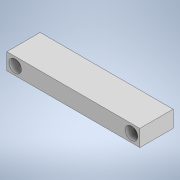
# Autodesk Inventor part: 3DPrintedFrameBackingPlate
Saved by Autodesk Inventor 2021 (Build 250183000, 183)
## iProperties
Created: 2021-10-26
Part Number: 3DPrintedFrameBackingPlate
Material: Generic
Document SubType Name: Sheet Metal
Designer: Unit-005
Density: 1 g/cm^3
Sheet Metal Rule: Default
Appearance: Default
Author: Unit-005
Autodesk Inventor part; units mm, degrees
ref_plane "YZ Plane" through (0, 0, 0) normal (1, 0, 0) x (0, 1, 0)
ref_plane "XZ Plane" through (0, 0, 0) normal (0, 1, 0) x (-1, 0, 0)
ref_plane "XY Plane" through (0, 0, 0) normal (0, 0, 1) x (1, 0, 0)
sketch "Sketch1" plane through (0, 0, 0) normal (0, 0, 1) x (1, 0, 0)
  line L0 (50.8, 6.35) -> (-50.8, 6.35)
  line L1 (-50.8, 6.35) -> (-50.8, -6.35)
  line L2 (-50.8, -6.35) -> (50.8, -6.35)
  line L3 (50.8, -6.35) -> (50.8, 6.35)
  line L4 (50.8, 6.35) -> (-50.8, -6.35) construction
  line L5 (-50.8, 6.35) -> (50.8, -6.35) construction
  point P0 (0, 0)
  dimension "d0" = 101.6
  dimension "d1" = 12.7
  constraints: 12 end point, 2 midpoint, 2 parallel, 1 horizontal, 1 perpendicular
  measures "d0" distance of L2.end L1.end
  measures "d1" distance of L1.end L0.end
extrude "Extrusion1" add sketch "Sketch1" against normal blind 25.4
sketch "Sketch2" plane through (0, 0, 0) normal (0, 0, 1) x (1, 0, 0)
  line L0 (-71.12, 0) -> (71.12, 0) projected
  line L1 (0, -8.89) -> (0, 8.89) projected
  line L2 (-50.8, 6.35) -> (-50.8, -6.35) projected
  line L3 (-50.8, -6.35) -> (50.8, -6.35) projected
  line L4 (50.8, -6.35) -> (50.8, 6.35) projected
  line L5 (50.8, 6.35) -> (-50.8, 6.35) projected
  point P0 (0, 0)
  point P1 (-44.45, 0)
  dimension "d5" = 44.45
  constraints: 1 point on line
  measures "d5" distance from line of L1 point (-44.45, 0)
hole "Hole1" at (-44.45, 0, 0) direction (0, 0, -1) diameter 6.35 end through all counterbore diameter 9.525 counterbore depth 6.35
mirror "Mirror1" about plane through (0, 0, 0) normal (1, 0, 0) of "Hole1"
equation "\"d11\" = Thickness"
equation "\"BendRadius\" = Thickness"
equation "\"BendReliefWidth\" = Thickness"
equation "\"BendReliefDepth\" = 0.5 * Thickness"
equation "\"CornerReliefSize\" = 4 * Thickness"
equation "\"MinimumRemnant\" = 2 * Thickness"
equation "\"TransitionRadius\" = BendRadius"
equation "\"JacobiRadiusSize\" = BendRadius"
equation "\"GapSize\" = Thickness"
equation "\"Thickness\" = 3.048"
body "Solid1"
